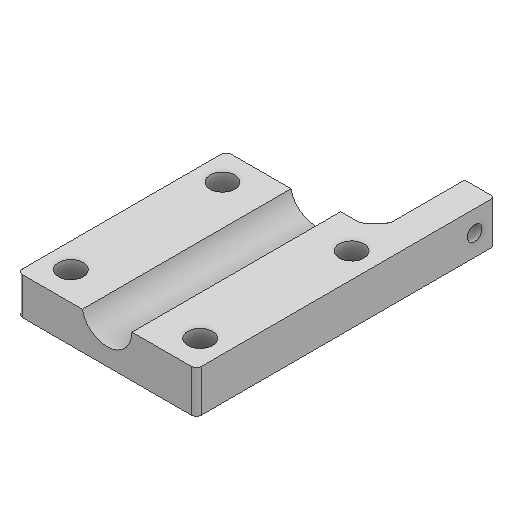
# Autodesk Inventor part: 3DP_ABS_X_Axis_Linear_Shaft_Clamp_Bottom_With_Endstop_Screw
Saved by Autodesk Inventor 2026.1 (Build 301233000, 233)
## iProperties
Created: 2017-05-25
Part Number: 3DP_ABS_X_Axis_Linear_Shaft_Clamp_Bottom_With_Endstop_Screw
Material: Ogólny
Document SubType Name: Modeling
Designer: Andrzej
Density: 1 g/cm^3
Appearance: Domyślna
Mass: 10.9619 g
Surface Area: 53.2605 cm^2
Volume: 10.9619 cm^3
Author: Andrzej
Autodesk Inventor part; units mm, degrees
ref_plane "YZ Plane" through (0, 0, 0) normal (1, 0, 0) x (0, 1, 0)
ref_plane "XZ Plane" through (0, 0, 0) normal (0, 1, 0) x (-1, 0, 0)
ref_plane "XY Plane" through (0, 0, 0) normal (0, 0, 1) x (1, 0, 0)
sketch "Szkic1" plane through (0, 0, 0) normal (0, 0, 1) x (1, 0, 0)
  line L0 (-10.3866, 5.557) -> (25.6134, 5.557)
  line L1 (25.6134, 5.557) -> (25.6134, -36.443)
  line L2 (25.6134, -36.443) -> (-10.3866, -36.443)
  line L3 (-10.3866, -36.443) -> (-10.3866, 5.557)
  point P0 (0, 0)
  point P1 (20.6134, -0.193)
  point P2 (20.6134, -30.693)
  point P3 (-5.3866, -0.193)
  point P4 (-5.3866, -30.693)
  dimension "d0" = 36
  dimension "d1" = 42
  dimension "d2" = 5
  dimension "d3" = 5
  dimension "d4" = 5
  dimension "d5" = 5
  dimension "d6" = 5.75
  dimension "d7" = 5.75
  dimension "d8" = 5.75
  dimension "d9" = 5.75
  constraints: 8 end point, 2 parallel, 1 horizontal, 1 perpendicular
  measures "d0" distance of L1.end L2.end
  measures "d1" distance of L0.end L1.end
  measures "d2" distance from line of L1 point (20.613, -0.193)
  measures "d3" distance from line of L1 point (20.613, -30.693)
  measures "d4" distance from line of L3 point (-5.387, -0.193)
  measures "d5" distance from line of L3 point (-5.387, -30.693)
  measures "d6" distance from line of L0 point (-5.387, -0.193)
  measures "d7" distance from line of L0 point (20.613, -0.193)
  measures "d8" distance from line of L2 point (20.613, -30.693)
  measures "d9" distance from line of L2 point (-5.387, -30.693)
extrude "Wyciągnięcie proste1" add sketch "Szkic1" along normal blind 7.5
hole "Otwór1" at (20.6134, -0.193, 0) at (20.6134, -30.693, 0) at (-5.3866, -0.193, 0) at (-5.3866, -30.693, 0) direction (0, 0, 1) diameter 5 end through all
sketch "Szkic2" plane through (-10.3866, -36.443, 0) normal (0, -1, 0) x (1, 0, 0)
  line L0 (36, 0) -> (0, 0) projected
  line L1 (36, 0) -> (36, 7.5) projected
  line L2 (0, 7.5) -> (36, 7.5) projected
  line L3 (0, 0) -> (0, 7.5) projected
  line L4 (36, 7.5) -> (0, 7.5) projected
  circle A0 centre (18, 8.5) radius 5.05
  point P0 (10.3866, 0)
  dimension "d19" = 36
  dimension "d25" = 8.5
  dimension "d26" = 18
  dimension "d27" = 10.1
  constraints: 1 centre point, 1 coincident
  measures "d19" distance between parallel lines of L1 L3
  measures "d25" distance from line of L0 point (18, 8.5)
  measures "d26" distance from line of L3 point (18, 8.5)
  measures "d27" diameter of A0
extrude "Wyciągnięcie proste2" cut sketch "Szkic2" against normal through all contours A0 L2 | L2 A0
sketch "Szkic3" plane through (0, 0, 7.5) normal (0, 0, 1) x (1, 0, 0)
  line L0 (25.6134, 5.557) -> (12.5634, 5.557) projected
  line L1 (12.5634, 5.557) -> (12.5634, -36.443) projected
  line L2 (-10.3866, -36.443) -> (2.6634, -36.443) projected
  line L3 (25.6134, -36.443) -> (25.6134, 5.557) projected
  circle A0 centre (20.6134, -0.193) radius 2.5 projected
  circle A1 centre (20.6134, -30.693) radius 2.5 projected
  line L4 (12.5634, -36.443) -> (25.6134, -36.443) projected
  line L5 (2.6634, -36.443) -> (2.6634, 5.557) projected
  line L6 (2.6634, 5.557) -> (-10.3866, 5.557) projected
  line L7 (-10.3866, 5.557) -> (-10.3866, -36.443) projected
  point P0 (0, 0)
extrude "Wyciągnięcie proste3" add sketch "Szkic3" along normal blind 1 contours L3 L4 L1 L0
sketch "Szkic4" plane through (0, 0, 0) normal (0, 0, -1) x (-1, 0, 0)
  circle A0 centre (5.3866, -0.193) radius 2.5 projected
  circle A1 centre (-20.6134, -0.193) radius 2.5 projected
  circle A2 centre (-20.6134, -30.693) radius 2.5 projected
  circle A3 centre (5.3866, -30.693) radius 2.5 projected
  line L0 (10.3866, 5.557) -> (-25.6134, 5.557) projected
  line L1 (-25.6134, 5.557) -> (-25.6134, -36.443) projected
  line L2 (-25.6134, -36.443) -> (10.3866, -36.443) projected
  line L3 (10.3866, -36.443) -> (10.3866, 5.557) projected
  line L4 (-25.6134, 5.557) -> (-25.6134, 23.557)
  line L5 (-25.6134, 23.557) -> (-19.6134, 23.557)
  line L6 (-19.6134, 23.557) -> (-19.6134, 5.557)
  point P0 (0, 0)
  dimension "d30" = 18
  dimension "d31" = 6
  constraints: 6 end point, 2 perpendicular, 1 point on line, 1 vertical
  measures "d30" distance of L5.end L6.end
  measures "d31" distance of L4.end L5.end
extrude "Wyciągnięcie proste4" add sketch "Szkic4" against normal blind 8.5 contours L0 L4 L5 L6
sketch "Szkic5" plane through (19.6134, 5.557, 0) normal (-1, 0, 0) x (0, 0, 1)
  line L0 (0, 0) -> (0, 18) projected
  line L1 (8.5, 0) -> (0, 0) projected
  line L2 (8.5, 18) -> (8.5, 0) projected
  line L3 (0, 18) -> (8.5, 18) projected
  point P0 (0, -5.557)
  point P1 (4.25, 14)
  dimension "d34" = 4.25
  dimension "d35" = 4
  dimension "d47" = 8.5
  measures "d34" distance from line of L2 point (4.25, 14)
  measures "d35" distance from line of L3 point (4.25, 14)
  measures "d47" distance of L0.end L2.start
hole "Otwór2" at (19.6134, 19.557, 4.25) direction (1, 0, 0) diameter 3 end through all
chamfer "Faza1" distance 3 angle 45 1 edges at (19.6134, 5.557, 4.25)
fillet "Zaokrąglenie2" radius 1 5 edges at (-10.3866, 5.557, 3.75) (-10.3866, -36.443, 3.75) (25.6134, -36.443, 4.25) (19.6134, 8.557, 4.25) (16.6134, 5.557, 4.25)
sketch "Szkic6" plane through (7.6134, -36.443, 8.5) normal (0, -1, 0) x (1, 0, 0)
  line L0 (17, 0) -> (17, -8.5) projected
  line L1 (4.95, 0) -> (17, 0) projected
  line L2 (4.95, -1) -> (4.95, 0) projected
  arc A0 (-4.95, -1) -> (4.95, -1) centre (0, 0) ccw projected
  line L3 (-17, -1) -> (-4.95, -1) projected
  line L4 (-17, -8.5) -> (-17, -1) projected
  line L5 (17, -8.5) -> (-17, -8.5) projected
  circle A1 centre (0, 0) radius 5.05
  point P0 (-7.6134, -8.5)
  dimension "d49" = 10.1
  constraints: 1 centre point, 1 coincident
  measures "d49" diameter of A1
extrude "Wyciągnięcie proste5" cut sketch "Szkic6" against normal through all contours A1 L2 L1 | L1 L2 A0 A1
fillet "Zaokrąglenie3" radius 0.5 2 edges at (19.6134, 23.557, 4.25) (25.6134, 23.557, 4.25)
equation "\"d7\" = d6"
equation "\"d8\" = d7"
equation "\"d9\" = d6"
equation "\"d26\" = 0.5 * d19"
equation "\"d34\" = 0.5 * d47"
